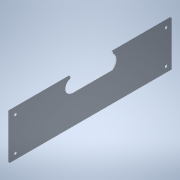
# Autodesk Inventor part: lc_box_side
Saved by Autodesk Inventor 2021.3 (Build 253353000, 353)
## iProperties
Created: 2019-07-19
Part Number: lc_box_side
Material: ポリカーボネート、クリア
Document SubType Name: Modeling
Designer: gisen
Density: 1.2 g/cm^3
Appearance: ポリカーボネート - クリア
Mass: 185.38 g
Surface Area: 1454.08 cm^2
Volume: 185.38 cm^3
Author: gisen
Autodesk Inventor part; units mm, degrees
ref_plane "YZ Plane" through (0, 0, 0) normal (1, 0, 0) x (0, 1, 0)
ref_plane "XZ Plane" through (0, 0, 0) normal (0, 1, 0) x (-1, 0, 0)
ref_plane "XY Plane" through (0, 0, 0) normal (0, 0, 1) x (1, 0, 0)
sketch "スケッチ1" plane through (0, 0, 0) normal (1, 0, 0) x (0, 1, 0)
  line L0 (125.6523, 179.1954) -> (45.6523, 179.1954)
  line L1 (45.6523, 179.1954) -> (45.6523, -110.8046)
  line L2 (45.6523, -110.8046) -> (125.6523, -110.8046)
  line L3 (125.6523, -110.8046) -> (125.6523, 179.1954)
  point P0 (0, 0)
  dimension "d0" = 80
  dimension "d1" = 290
  constraints: 8 end point, 2 parallel, 1 horizontal, 1 perpendicular
  measures "d0" distance of L0.start L0.end
  measures "d1" distance of L2.end L0.start
extrude "押し出し1" add sketch "スケッチ1" along normal blind 2.6
sketch "スケッチ2" plane through (2.6, 0, 0) normal (1, 0, 0) x (0, 0, -1)
  line L0 (-179.1954, 125.6523) -> (-179.1954, 45.6523) projected
  line L1 (-179.1954, 45.6523) -> (110.8046, 45.6523) projected
  line L2 (110.8046, 45.6523) -> (110.8046, 125.6523) projected
  line L3 (110.8046, 125.6523) -> (-179.1954, 125.6523) projected
  line L4 (-34.1954, 85.6523) -> (-34.1954, 125.6523)
  line L5 (110.8046, 125.6523) -> (-179.1954, 125.6523) projected
  line L6 (-34.1954, 85.6523) -> (110.8046, 85.6523)
  point P0 (0, 0)
  point P1 (-169.1954, 115.6523)
  point P2 (100.8046, 115.6523)
  point P3 (-169.1954, 55.6523)
  point P4 (100.8046, 55.6523)
  dimension "d4" = 10
  dimension "d5" = 10
  constraints: 4 end point, 3 symmetric about line, 2 midpoint
  measures "d4" distance from line of L3 point (-169.195, 115.652)
  measures "d5" distance from line of L0 point (-169.195, 115.652)
hole "穴1" at (2.6, 115.6523, 169.1954) at (2.6, 115.6523, -100.8046) at (2.6, 55.6523, 169.1954) at (2.6, 55.6523, -100.8046) direction (-1, 0, 0) diameter 4.5 depth 10 tip angle 118
sketch "スケッチ4" plane through (0, 0, 0) normal (-1, 0, 0) x (0, 0, 1)
  ellipse E0 centre (2.4593, 110.6523) end of major axis (2.4593, 125.1521) minor radius 14.4996 (-5.7266, 122.6204) -> (-6.1243, 98.9661) ccw projected
  line L0 (-5.7266, 125.6523) -> (-5.7266, 122.6204) projected
  line L1 (-4.4935, 97.7683) -> (66.6998, 97.7683) projected
  line L2 (66.6998, 97.7683) -> (70.683, 98.6842) projected
  ellipse E1 centre (67.383, 110.6523) end of major axis (67.383, 123.067) minor radius 12.4145 (70.683, 98.6842) -> (70.683, 122.6204) ccw projected
  line L3 (70.683, 122.6204) -> (70.683, 125.6523) projected
  ellipse E2 centre (67.383, 110.6523) end of major axis (67.383, 123.067) minor radius 12.4145 (70.683, 98.6842) -> (70.683, 122.6204) ccw projected
  line L4 (-6.1243, 98.9661) -> (-4.4935, 97.7683) projected
  line L5 (-110.8046, 125.6523) -> (179.1954, 125.6523) projected
  arc A0 (66.6955, 101.0165) -> (66.6955, 120.2881) centre (66.6954, 110.6523) ccw projected
  arc A1 (1.6954, 120.1437) -> (1.6954, 101.1609) centre (1.6954, 110.6523) ccw projected
  line L6 (1.6954, 120.1437) -> (66.6955, 120.2881)
  line L7 (66.6955, 101.0165) -> (1.6954, 101.1609)
  line L8 (1.6954, 120.1437) -> (1.6954, 125.6523)
  line L9 (-110.8046, 125.6523) -> (179.1954, 125.6523) projected
  line L10 (66.6955, 120.2881) -> (66.6955, 125.6523)
  point P0 (0, 0)
  constraints: 8 end point, 2 perpendicular, 2 point on line, 3 other
extrude "押し出し3" cut sketch "スケッチ4" against normal through all
